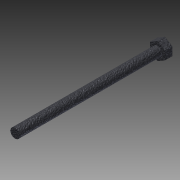
# Autodesk Inventor part: quarter-inch-rod
Saved by Autodesk Inventor 2014 (Build 180170000, 170)
## iProperties
Created: 2013-11-06
Part Number: quarter-inch-rod
Material: Iron, Cast
Document SubType Name: Modeling
Designer: stephen
Density: 1 g/cm^3
Appearance: Iron - Cast
Author: stephen
Autodesk Inventor part; units mm, degrees
ref_plane "YZ Plane" through (0, 0, 0) normal (1, 0, 0) x (0, 1, 0)
ref_plane "XZ Plane" through (0, 0, 0) normal (0, 1, 0) x (-1, 0, 0)
ref_plane "XY Plane" through (0, 0, 0) normal (0, 0, 1) x (1, 0, 0)
sketch "Sketch1" plane through (0, 0, 0) normal (0, 0, 1) x (1, 0, 0)
  circle A0 centre (0, 0) radius 2.5
  line L0 (1.3379, -2.1119) -> (1.34, -2.1119)
  point P0 (-1.3379, -2.1119)
  dimension "d0" = 5
  constraints: 2 end point, 2 point on circle, 1 centre point, 1 coincident, 1 horizontal
  measures "d0" diameter of A0
extrude "Extrusion1" add sketch "Sketch1" along normal blind 80
sketch "Sketch2" plane through (0, 0, 0) normal (0, 0, -1) x (-1, 0, 0)
  circle A0 centre (0, 0) radius 2.5 projected
  line L0 (0, -4.6188) -> (-4, -2.3094)
  line L1 (-4, -2.3094) -> (-4, 2.3094)
  line L2 (-4, 2.3094) -> (0, 4.6188)
  line L3 (0, 4.6188) -> (4, 2.3094)
  line L4 (4, 2.3094) -> (4, -2.3094)
  line L5 (4, -2.3094) -> (0, -4.6188)
  dimension "d4" = 8
  constraints: 12 end point, 1 coincident, 13 other
  measures "d4" distance between parallel lines of L4 L1
extrude "Extrusion2" add sketch "Sketch2" against normal blind 4
body "Solid1"
